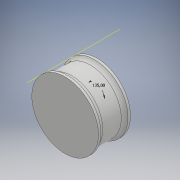
# Autodesk Inventor part: Kolo_silnik
Saved by Autodesk Inventor 2018 (Build 220112000, 112)
## iProperties
Created: 2019-08-04
Part Number: Kolo_silnik
Material: Ogólny
Document SubType Name: Modeling
Designer: Raven
Density: 1 g/cm^3
Appearance: Domyślna
Author: Raven
Autodesk Inventor part; units mm, degrees
ref_plane "YZ Plane" through (0, 0, 0) normal (1, 0, 0) x (0, 1, 0)
ref_plane "XZ Plane" through (0, 0, 0) normal (0, 1, 0) x (-1, 0, 0)
ref_plane "XY Plane" through (0, 0, 0) normal (0, 0, 1) x (1, 0, 0)
sketch "Szkic1" plane through (0, 0, 0) normal (0, 0, 1) x (1, 0, 0)
  line L0 (0, 0) -> (13.5, 0)
  line L1 (13.5, 0) -> (13.5, 1)
  line L2 (13.5, 1) -> (12.5, 1)
  line L3 (12.5, 1) -> (12.5, 12)
  line L4 (12.5, 12) -> (13.5, 12)
  line L5 (13.5, 12) -> (13.5, 13)
  line L6 (13.5, 13) -> (5.5, 13)
  line L7 (5.5, 13) -> (0, 13)
  line L8 (0, 13) -> (0, 0)
  dimension "d0" = 13.5
  dimension "d1" = 1
  dimension "d2" = 1
  dimension "d3" = 11
  dimension "d4" = 1
  dimension "d5" = 1
  dimension "d6" = 8
  constraints: 18 end point, 6 perpendicular, 2 horizontal, 1 vertical
  measures "d0" distance of L0.start L0.end
  measures "d1" distance of L0.end L1.end
  measures "d2" distance of L1.end L2.end
  measures "d3" distance of L2.end L3.end
  measures "d4" distance of L3.end L4.end
  measures "d5" distance of L4.end L5.end
  measures "d6" distance of L5.end L6.end
revolve "Obrót1" add sketch "Szkic1" angle 360 about axis through (0, 13, 0) along (0, -1, 0)
sketch "Szkic2" plane through (0, 13, 0) normal (0, 1, 0) x (1, 0, 0)
  line L0 (0, 0) -> (-2, 0) construction
  line L1 (0, 0) -> (2, 0) construction
  line L2 (0, 0) -> (0, 2) construction
  line L3 (0, 0) -> (0, -2) construction
  line L4 (0, 2) -> (-0.8, 2) construction
  line L5 (0, 2) -> (0.8, 2) construction
  line L6 (2, 0) -> (2, 0.8) construction
  line L7 (2, 0) -> (2, -0.8) construction
  line L8 (0, -2) -> (0.8, -2) construction
  line L9 (0, -2) -> (-0.8, -2) construction
  line L10 (-2, 0) -> (-2, 0.8) construction
  line L11 (-2, 0) -> (-2, -0.8) construction
  line L12 (-2, -0.8) -> (-2, 0.8)
  line L13 (-2, 0.8) -> (-0.8, 0.8)
  line L14 (-0.8, 0.8) -> (-0.8, 2)
  line L15 (-0.8, 2) -> (0.8, 2)
  line L16 (0.8, 2) -> (0.8, 0.8)
  line L17 (0.8, 0.8) -> (2, 0.8)
  line L18 (2, 0.8) -> (2, -0.8)
  line L19 (2, -0.8) -> (0.8, -0.8)
  line L20 (0.8, -0.8) -> (0.8, -2)
  line L21 (0.8, -2) -> (-0.8, -2)
  line L22 (-0.8, -2) -> (-0.8, -0.8)
  line L23 (-0.8, -0.8) -> (-2, -0.8)
  dimension "d12" = 0.8
  dimension "d13" = 2
  dimension "d14" = 2
  dimension "d15" = 2
  dimension "d16" = 2
  dimension "d17" = 0.8
  dimension "d18" = 0.8
  dimension "d19" = 0.8
  constraints: 48 end point, 7 horizontal, 7 vertical, 6 perpendicular, 4 point on line, 3 collinear
  measures "d12" distance of L0.end L11.end
  measures "d13" distance of L0.start L3.end
  measures "d14" distance of L0.start L2.end
  measures "d15" distance of L0.start L0.end
  measures "d16" distance of L0.start L1.end
  measures "d17" distance of L0.end L10.end
  measures "d18" distance of L2.end L4.end
  measures "d19" distance of L2.end L5.end
extrude "Wyciągnięcie proste1" cut sketch "Szkic2" against normal blind 2
sketch "Szkic3" plane through (0, 11, 0) normal (0, 1, 0) x (1, 0, 0)
  circle A0 centre (0, 0) radius 0.9
  dimension "d22" = 1.8
  constraints: 1 centre point, 1 coincident
  measures "d22" diameter of A0
extrude "Wyciągnięcie proste2" cut sketch "Szkic3" against normal blind 1
sketch "Szkic4" plane through (0, 13, 0) normal (0, 1, 0) x (1, 0, 0)
  line L0 (-0.8, -2) -> (-0.8, -0.8) construction
  line L1 (-0.8, -0.8) -> (-9.5459, -9.5459) construction
  circle A0 centre (0, 0) radius 13.5 construction
  line L2 (-0.8, -0.8) -> (11.5686, -0.8) construction
  dimension "d25" = 135
  constraints: 4 end point, 1 equal length, 1 horizontal, 2 other
  measures "d25" angle of L1 L2
ref_plane "Płaszczyzna konstrukcyjna1" through (-9.5459, 13, 9.5459) normal (-0.7071068, 0, 0.7071068) x (0, -1, 0)
sketch "Szkic5" plane through (-9.5459, 13, 9.5459) normal (-0.7071068, 0, 0.7071068) x (0, -1, 0)
  line L0 (0, 0) -> (2, 0) construction
  line L1 (0, 0) -> (2, 0) construction
  line L2 (2, 0) -> (3, 0) construction
  line L3 (3, -0.9) -> (3, 0.9) construction
  circle A0 centre (3, 0) radius 1
  point P0 (13, 0)
  dimension "d26" = 2
  constraints: 4 end point, 1 centre point, 1 coincident, 1 collinear, 1 midpoint
  measures "d26" diameter of A0
extrude "Wyciągnięcie proste3" cut sketch "Szkic5" against normal blind 12.75
fillet "Zaokrąglenie1" radius 2 2 edges at (-12.5, 1, 0) (-12.5, 12, 0)
equation "\"d14\" = d13"
equation "\"d15\" = d13"
equation "\"d16\" = d13"
equation "\"d17\" = d12"
equation "\"d18\" = d12"
equation "\"d19\" = d12"
